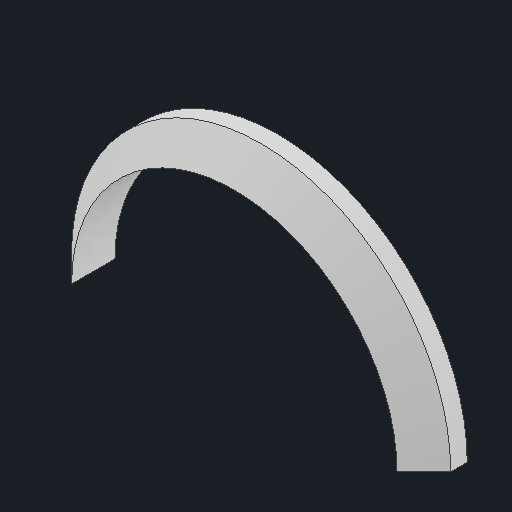
# Autodesk Inventor part: Venstre_bearing_lock
Saved by Autodesk Inventor 2026.1 (Build 301233020, 233B)
## iProperties
Created: 2025-09-28
Part Number: Venstre_bearing_lock
Material: Generic
Document SubType Name: Modeling
Designer: Malthe Sennels
Density: 1 g/cm^3
Appearance: Default
Author: Malthe Sennels
Autodesk Inventor part; units mm, degrees
ref_plane "YZ Plane" through (0, 0, 0) normal (1, 0, 0) x (0, 1, 0)
ref_plane "XZ Plane" through (0, 0, 0) normal (0, 1, 0) x (-1, 0, 0)
sketch "Sketch1" plane through (0, 0, 0) normal (0, 0, 1) x (1, 0, 0)
  arc A0 (21.2, 0) -> (-21.2, 0) centre (0, 0) ccw projected
  circle A1 centre (0, 0) radius 12.5 projected
  circle A2 centre (0, 0) radius 11
  line L0 (-18.2, -70.4538) -> (-18.2, -81.7961) projected
  line L1 (-17.25, -10.1789) -> (-12.75, -10.1789) projected
  line L2 (-12.75, -10.1789) -> (-12.75, -5.6789) projected
  line L3 (-12.75, -5.6789) -> (-17.25, -5.6789) projected
  arc A3 (18.2, 0) -> (-18.2, 0) centre (0, 0) ccw projected
  line L4 (18.2, -67.8385) -> (18.2, -39.4538) projected
  line L5 (17.25, -5.6789) -> (12.75, -5.6789) projected
  line L6 (12.75, -5.6789) -> (12.75, -10.1789) projected
  line L7 (12.75, -10.1789) -> (17.25, -10.1789) projected
  circle A4 centre (0, -53.6461) radius 2.5 projected
  line L8 (-18.2, -81.7961) -> (18.2, -81.7961) projected
  line L9 (-17.25, -5.6789) -> (-17.25, -10.1789) projected
  line L10 (17.25, -10.1789) -> (17.25, -5.6789) projected
  line L11 (-18.2, 0) -> (-21.2, 0) projected
  arc A5 (18.2, 0) -> (-18.2, 0) centre (0, 0) ccw projected
  line L12 (21.2, 0) -> (18.2, 0) projected
  arc A6 (-18.2, -70.4538) -> (-18.2, -67.8385) centre (-15.5, -69.1461) ccw projected
  line L13 (-18.2, -39.4538) -> (-18.2, -67.8385) projected
  arc A7 (-18.2, -39.4538) -> (-18.2, -36.8385) centre (-15.5, -38.1461) ccw projected
  line L14 (-18.2, 0) -> (-18.2, -36.8385) projected
  line L15 (18.2, -36.8385) -> (18.2, 0) projected
  arc A8 (18.2, -36.8385) -> (18.2, -39.4538) centre (15.5, -38.1461) ccw projected
  arc A9 (18.2, -67.8385) -> (18.2, -70.4538) centre (15.5, -69.1461) ccw projected
  line L16 (18.2, -81.7961) -> (18.2, -70.4538) projected
  point P0 (0, 0)
  point P1 (0, 0)
  constraints: 1 centre point, 2 other
ref_plane "Work Plane1" through (-15, -65, 4.85) normal (0, 0, 1) x (1, 0, 0)
extrude "Extrusion1" add sketch "Sketch1" along normal up to surface (4.85 mm away) contours L12 A3 L11 A0
chamfer "Chamfer1" distance 3 angle 45 1 edges at (0, 21.2, 4.85)
chamfer "Chamfer2" [suppressed]
sketch "Sketch2" plane through (-12, -18, 4.85) normal (0, 0, 1) x (1, 0, 0)
  circle A0 centre (27, 10.0711) radius 1.75 projected
  circle A1 centre (-3, 10.0711) radius 1.75 projected
  point P0 (12, 18)
extrude "Extrusion2" cut sketch "Sketch2" against normal through all
sketch "Sketch3" plane through (-12, -18, 4.85) normal (0, 0, 1) x (1, 0, 0)
  circle A0 centre (-3, 10.0711) radius 1.75 projected
  circle A1 centre (-3, 10.0711) radius 3
  arc A2 (27, 11.8211) -> (27, 8.3211) centre (27, 10.0711) ccw projected
  circle A3 centre (27, 10.0711) radius 3
  point P0 (12, 18)
  dimension "d10" = 6
  dimension "d11" = 6
  constraints: 2 centre point, 2 coincident
  measures "d10" diameter of A1
  measures "d11" diameter of A3
extrude "Extrusion3" cut sketch "Sketch3" against normal blind 2 contours A0 | A1 | A3
sketch "Sketch4" plane through (0, 0, 0) normal (1, 0, 0) x (0, 1, 0)
  arc A0 (11, -2.3164) -> (13.125, 0) centre (10.8, 0) ccw
  circle A1 centre (10.8, 0) radius 2.325
  line L0 (0, -21.9803) -> (0, 17.051)
  point P0 (0, 0)
  point P1 (13.125, 0)
  constraints: 2 end point, 2 point on circle, 1 centre point, 1 coincident, 1 vertical, 7 other
revolve "Revolution1" cut sketch "Sketch4" angle 360 about axis through (0, 0, -21.9803) along (0, 0, 1)
body "Solid1"
